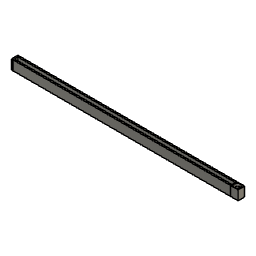
board_edge v12 (Autodesk Fusion 360 design; units mm, degrees)
Autodesk Fusion 360 part; units mm, degrees
sketch "Esquisse1" plane through (0, 0, 0) normal (0, 0, 1) x (1, 0, 0) in component "edge"
  line L0 (14.9828, 0) -> (129.9828, 0)
  line L1 (129.9828, 0) -> (129.9828, -0.8)
  line L2 (129.9828, -0.8) -> (14.9828, -0.8)
  line L3 (14.9828, -0.8) -> (14.9828, 0)
  line L4 (14.9828, 0) -> (129.9828, 0)
  line L5 (129.9828, 0) -> (129.9828, 1.8)
  line L6 (129.9828, 1.8) -> (14.9828, 1.8)
  line L7 (14.9828, 1.8) -> (14.9828, 0)
  line L8 (14.9828, 1.8) -> (129.9828, 1.8)
  line L9 (129.9828, 1.8) -> (129.9828, 2.6)
  line L10 (129.9828, 2.6) -> (14.9828, 2.6)
  line L11 (14.9828, 2.6) -> (14.9828, 1.8)
  line L12 (129.9828, -0.8) -> (133.9828, -0.8)
  line L13 (133.9828, -0.8) -> (133.9828, 2.6)
  line L14 (133.9828, 2.6) -> (129.9828, 2.6)
  line L15 (129.9828, 2.6) -> (129.9828, -0.8)
  line L16 (14.9828, -0.8) -> (14.1828, -0.8)
  line L17 (14.1828, -0.8) -> (14.1828, 2.6)
  line L18 (14.1828, 2.6) -> (14.9828, 2.6)
  line L19 (14.9828, 2.6) -> (14.9828, -0.8)
  line L20 (129.9828, -0.8) -> (133.9828, 2.6) construction
  line L21 (133.9828, -0.8) -> (129.9828, 2.6) construction
  circle A0 centre (131.9828, 0.9) radius 0.7
  dimension "EdgePhotoLen" = 115
  dimension "d2" = 0.8
  dimension "d3" = 1.8
  dimension "d4" = 115
  dimension "d5" = 0.8
  dimension "d10" = 4
  dimension "d11" = 0.8
  dimension "d14" = 1.4
  constraint horizontal L0
  constraint vertical L1
  constraint horizontal L2
  constraint vertical L3
  constraint horizontal L4
  constraint vertical L5
  constraint horizontal L6
  constraint vertical L7
  constraint horizontal L8
  constraint vertical L9
  constraint horizontal L10
  constraint vertical L11
  constraint horizontal L12
  constraint vertical L13
  constraint horizontal L14
  constraint vertical L15
  constraint horizontal L16
  constraint vertical L17
  constraint horizontal L18
  constraint vertical L19
  constraint midpoint L21 A0.centre
  measures "EdgePhotoLen" distance of L0.start L0.end
  measures "d2" distance of L0.start L2.end
  measures "d3" distance of L0.start L6.end
  measures "d4" distance of L6.end L5.end
  measures "d5" distance of L6.end L10.end
  measures "d10" distance of L1.end L12.end
  measures "d11" distance of L2.end L16.end
  measures "d14" diameter of A0
extrude "Extrusion1" add sketch "Esquisse1" along normal blind 0.8 contours L0 L4 L5 L6 L7 L8 L15 L19 makes body 1 in component "edge"
extrude "Extrusion2" add sketch "Esquisse1" along normal blind 5 separate body contours L0 L1 L2 L3 L4 L15 L19 | L6 L8 L9 L10 L11 L15 L19 makes body 2 at (91.6495, 2.6, 1.6667) makes body 3 at (53.3161, 0, 1.6667) in component "edge"
extrude "Extrusion3" add sketch "Esquisse1" along normal blind 5 separate body contours L3 L7 L11 L16 L17 L18 L19 | L1 L5 L9 L12 L13 L14 L15 | A0 makes body 4 at (14.9828, 0.3333, 1.6667) makes body 5 at (131.3161, -0.8, 1.6667) in component "edge"
sketch "Esquisse3" plane through (0, 0, 5) normal (0, 0, 1) x (-1, 0, 0)
  line L0 (-129.9828, -2.6) -> (-129.9828, 0.8)
  line L1 (-129.9828, 0.8) -> (-133.9828, 0.8)
  line L2 (-133.9828, 0.8) -> (-133.9828, -2.6)
  line L3 (-133.9828, -2.6) -> (-129.9828, -2.6)
  line L4 (-129.9828, -2.6) -> (-133.9828, 0.8) construction
  line L5 (-129.9828, 0.8) -> (-133.9828, -2.6) construction
  point P0 (-131.9828, -0.9)
  constraint coincident L0.start L3.end
  constraint coincident L1.end L2.start
  constraint coincident L0.end L1.start
  constraint coincident L2.end L3.start
  constraint midpoint L5 P0
hole "Perçage2" at (131.9828, 0.9, 5) direction (0, 0, -1) diameter 1.221 depth 8 tip angle 180 countersink diameter 3.1 countersink angle 90 bodies 5 in component "edge"
thread "Filetage2" "ISO Metric profile 1.4 M1.4x0.3 6H" thread offset 0 thread depth 7.4 in component "edge"
sketch "Esquisse4" plane through (0, 0, 5) normal (0, 0, 1) x (-1, 0, 0)
  circle A0 centre (-131.9828, -0.9) radius 1.55
  line L0 (-129.9828, -2.6) -> (-129.9828, 0.8)
  line L1 (-129.9828, 0.8) -> (-133.9828, 0.8)
  line L2 (-133.9828, 0.8) -> (-133.9828, -2.6)
  line L3 (-133.9828, -2.6) -> (-129.9828, -2.6)
  circle A1 centre (-131.9828, -0.9) radius 0.8363
  constraint concentric A0 A1
extrude "Extrusion6" cut sketch "Esquisse4" against normal blind 2 contours A1 bodies 5 in component "edge"
component "edge" placed x (1, 0, 0) y (0, 1, 0) z (0, 0, 1) at (0, 0, 0)
equation "d4 = EdgePhotoLen"
